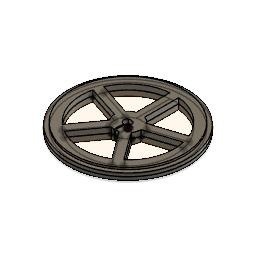
_Wheel.690aa9d6-0443-4a5d-b359-7cdf34e08d0b (Autodesk Fusion 360 design; units mm, degrees)
Autodesk Fusion 360 part; units mm, degrees
sketch "Sketch1" plane through (0, 0, 0) normal (0, 1, 0) x (1, 0, 0)
  circle A0 centre (0, 0) radius 45
  circle A1 centre (0, 0) radius 2.95
  line L0 (-1.9653, 2.2) -> (1.9653, 2.2)
  circle A2 centre (0, 0) radius 35
  circle A3 centre (0, 0) radius 10
  line L1 (-3.25, 34.8488) -> (-3.25, 9.4571)
  line L2 (3.25, 34.8488) -> (3.25, 9.4571)
  line L3 (-34.1475, 7.6779) -> (-9.9986, -0.1685)
  line L4 (-32.1389, 13.8598) -> (-7.99, 6.0134)
  line L5 (-17.8543, -30.1036) -> (-2.9295, -9.5613)
  line L6 (-23.1129, -26.283) -> (-8.1881, -5.7407)
  line L7 (23.1129, -26.283) -> (8.1881, -5.7407)
  line L8 (17.8543, -30.1036) -> (2.9295, -9.5613)
  line L9 (32.1389, 13.8598) -> (7.99, 6.0134)
  line L10 (34.1475, 7.6779) -> (9.9986, -0.1685)
  line L11 (-0.5, -2.9073) -> (-0.5, -9.9875)
  line L12 (0.5, -2.9073) -> (0.5, -9.9875)
  circle A4 centre (0, 0) radius 42
  dimension "d1" = 90
  dimension "d2" = 5.9
  dimension "d3" = 2.2
  dimension "d4" = 70
  dimension "d5" = 20
  dimension "d6" = 6.5
  dimension "d8" = 360
  dimension "d9" = 1
  dimension "d10" = 84
  dimension "d25" = 25.3916
  dimension "d26" = 20
  measures "d1" diameter of A0
  measures "d2" diameter of A1
  measures "d3" distance of A0.centre L0
  measures "d4" diameter of A2
  measures "d5" diameter of A3
  measures "d6" distance of L1 L2
  measures "d9" distance of L11 L12
  measures "d10" diameter of A4
  measures "d25" distance of L10.start L10.end
  measures "d26" diameter of A3
extrude "Extrude1" add sketch "Sketch1" along normal mid plane 5 contours A0
extrude "Extrude2" add sketch "Sketch1" along normal mid plane 8 contours A4
extrude "Extrude6" add sketch "Sketch1" along normal mid plane 8 contours A1 A3 L11 L12 | A1 L0 | A2 A3 L7 L8 | A2 A3 L5 L6 | A2 A3 L9 L10 | A2 A3 L3 L4 | A2 A3 L1 L2 picked at (5.7516, 5.0158) picked at (-0.1692, 2.4959)
extrude "Extrude7" add sketch "Sketch1" along normal blind 4 contours A1 A3 L11 L12 | A1 L0 picked at (5.7516, 5.0158) picked at (-0.1692, 2.4959)
